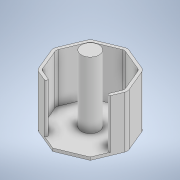
# Autodesk Inventor part: holder-8
Saved by Autodesk Inventor 2020 (Build 240168000, 168)
## iProperties
Created: 2020-02-16
Part Number: holder-8
Material: Generic
Document SubType Name: Modeling
Designer: Ball
Density: 1 g/cm^3
Appearance: Default
Author: Ball
Autodesk Inventor part; units mm, degrees
ref_plane "YZ Plane" through (0, 0, 0) normal (1, 0, 0) x (0, 1, 0)
ref_plane "XZ Plane" through (0, 0, 0) normal (0, 1, 0) x (-1, 0, 0)
ref_plane "XY Plane" through (0, 0, 0) normal (0, 0, 1) x (1, 0, 0)
sketch "Sketch1" plane through (0, 0, 0) normal (0, 1, 0) x (-1, 0, 0)
  line L0 (54.9855, 0) -> (38.8806, -38.8806)
  line L1 (38.8806, -38.8806) -> (0, -54.9855)
  line L2 (0, -54.9855) -> (-38.8806, -38.8806)
  line L3 (-38.8806, -38.8806) -> (-54.9855, 0)
  line L4 (-54.9855, 0) -> (-38.8806, 38.8806)
  line L5 (-38.8806, 38.8806) -> (0, 54.9855)
  line L6 (0, 54.9855) -> (38.8806, 38.8806)
  line L7 (38.8806, 38.8806) -> (54.9855, 0)
  point P0 (0, 0)
  dimension "d0" = 50.8
  constraints: 16 end point, 1 other
  measures "d0" distance from line of L0 point (0, 0)
extrude "Extrusion1" add sketch "Sketch1" along normal blind 76.2
sketch "Sketch2" plane through (0, 76.2, 0) normal (0, 1, 0) x (1, 0, 0)
  line L0 (-50.3667, 0) -> (-35.6147, 35.6147)
  line L1 (-35.6147, 35.6147) -> (0, 50.3667)
  line L2 (0, 50.3667) -> (35.6147, 35.6147)
  line L3 (35.6147, 35.6147) -> (50.3667, 0)
  line L4 (50.3667, 0) -> (35.6147, -35.6147)
  line L5 (35.6147, -35.6147) -> (0, -50.3667)
  line L6 (0, -50.3667) -> (-35.6147, -35.6147)
  line L7 (-35.6147, -35.6147) -> (-50.3667, 0)
  line L8 (38.8806, -38.8806) -> (54.9855, 0) projected
  point P0 (0, 0)
  point P1 (0, 0)
  dimension "d4" = 4.2672
  constraints: 16 end point, 1 coincident, 17 other
  measures "d4" distance between parallel lines of L8 L4
extrude "Extrusion2" cut sketch "Sketch2" against normal blind 71.9328
sketch "Sketch3" plane through (0, 76.2, 0) normal (0, 1, 0) x (1, 0, 0)
  line L0 (-35.6147, -35.6147) -> (-50.3667, 0) projected
  line L1 (-38.8806, -38.8806) -> (0, -54.9855) projected
  line L2 (-32.6208, -74.0252) -> (-0.337, -89.435)
  line L3 (50.3667, 0) -> (35.6147, -35.6147) projected
  line L4 (0, -54.9855) -> (38.8806, -38.8806) projected
  line L5 (63.1414, -63.1414) -> (-0.337, -89.435)
  line L6 (0, -50.3667) -> (-35.6147, -35.6147) projected
  line L7 (-17.8073, -42.9907) -> (-32.6208, -74.0252)
  line L8 (35.6147, 35.6147) -> (50.3667, 0) projected
  line L9 (54.9855, 0) -> (38.8806, 38.8806) projected
  line L10 (82.5817, -31.5707) -> (63.1414, -63.1414)
  line L11 (42.9907, -17.8073) -> (82.5817, -31.5707)
  line L12 (-17.8073, -42.9907) -> (42.9907, -17.8073)
  point P0 (0, 0)
  constraints: 12 end point, 2 midpoint, 1 parallel, 1 perpendicular
extrude "Extrusion3" cut sketch "Sketch3" against normal blind 71.9328
fillet "Fillet1" radius 2.1336 4 edges at (-17.8073, 40.2336, 42.9907) (-19.648, 40.2336, 46.847) (42.9907, 40.2336, 17.8073) (47.0281, 40.2336, 19.2109)
sketch "Sketch4" plane through (0, 4.2672, 0) normal (0, 1, 0) x (1, 0, 0)
  circle A0 centre (0, 0) radius 12.954
  dimension "d10" = 25.908
  constraints: 1 centre point, 1 coincident
  measures "d10" diameter of A0
extrude "Extrusion4" add sketch "Sketch4" along normal blind 97.3328
fillet "Fillet2" radius 6.35 6 edges at (-50.3667, 40.2336, 0) (-35.6147, 40.2336, -35.6147) (0, 40.2336, -50.3667) (35.6147, 40.2336, -35.6147) (50.3667, 40.2336, 0) (-35.6147, 40.2336, 35.6147)
fillet "Fillet3" radius 8.89 6 edges at (54.9855, 38.1, 0) (38.8806, 38.1, -38.8806) (-38.8806, 38.1, 38.8806) (-54.9855, 38.1, 0) (-38.8806, 38.1, -38.8806) (0, 38.1, -54.9855)
body "Solid1"
